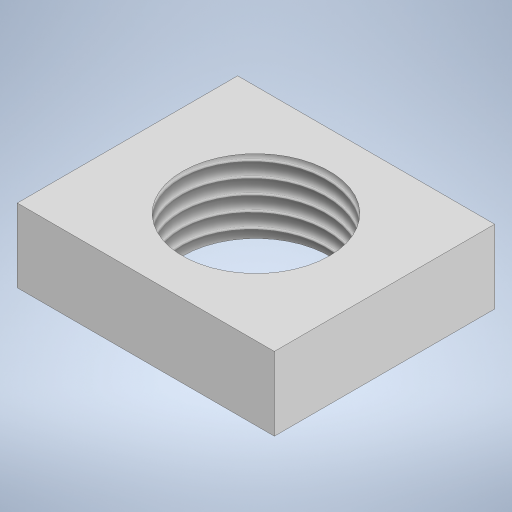
# Autodesk Inventor part: Деталь перемещение по резьбе
Saved by Autodesk Inventor 2023 (Build 270158000, 158)
## iProperties
Created: 2022-04-28
Part Number: Деталь перемещение по резьбе
Material: Типовые
Document SubType Name: Modeling
Designer: User
Density: 1 g/cm^3
Appearance: По умолчанию
Author: User
Autodesk Inventor part; units mm, degrees
ref_plane "YZ Plane" through (0, 0, 0) normal (1, 0, 0) x (0, 1, 0)
ref_plane "XZ Plane" through (0, 0, 0) normal (0, 1, 0) x (-1, 0, 0)
ref_plane "XY Plane" through (0, 0, 0) normal (0, 0, 1) x (1, 0, 0)
sketch "Эскиз1" plane through (0, 0, 0) normal (0, 1, 0) x (-1, 0, 0)
  line L0 (0, 0) -> (-35, 0)
  line L1 (-35, 0) -> (-35, 30)
  line L2 (-35, 30) -> (0, 30)
  line L3 (0, 30) -> (0, 0)
  line L4 (-17.5, 25) -> (-17.5, 0)
  line L5 (-17.5, 25) -> (-17.5, 15)
  circle A0 centre (-17.5, 15) radius 10
  dimension "d0" = 35
  dimension "d1" = 30
  dimension "d17" = 10
  dimension "d20" = 15
  constraints: 12 end point, 2 parallel, 1 coincident, 1 horizontal, 1 midpoint, 1 perpendicular, 1 point on line, 1 vertical alignment, 2 other
  measures "d0" distance of L1.end L2.end
  measures "d1" distance of L0.end L1.end
  measures "d17" distance of L4.start L5.end
  measures "d20" distance of L4.end L5.end
extrude "Выдавливание1" add sketch "Эскиз1" along normal blind 10
thread "Резьба2" size "M20x2" class "6H" standard "ISO Metric profile" full length
